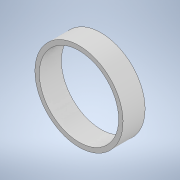
# Autodesk Inventor part: 轴承盖挡圈
Saved by Autodesk Inventor 2020 (Build 240168000, 168)
## iProperties
Created: 2021-06-16
Part Number: 轴承盖挡圈
Material: 常规
Document SubType Name: Modeling
Designer: dell
Density: 1 g/cm^3
Appearance: 默认
Author: dell
Autodesk Inventor part; units mm, degrees
ref_plane "YZ Plane" through (0, 0, 0) normal (1, 0, 0) x (0, 1, 0)
ref_plane "XZ Plane" through (0, 0, 0) normal (0, 1, 0) x (-1, 0, 0)
ref_plane "工作平面1" through (-16.8643, 32.5395, 28) normal (0, 0, 1) x (-0.4601, 0.8878, 0)
sketch "草图1" plane through (-16.8643, 32.5395, 28) normal (0, 0, 1) x (-0.4601, 0.8878, 0)
  circle A0 centre (-36.65, 0) radius 65 construction
  circle A1 centre (-36.65, 0) radius 40
  circle A2 centre (-36.65, 0) radius 32
  point P0 (-36.65, 0)
  dimension "d0" = 80
  dimension "d1" = 64
  constraints: 2 centre point, 2 coincident
  measures "d0" diameter of A1
  measures "d1" diameter of A2
extrude "拉伸1" add sketch "草图1" along normal blind 20
sketch "草图2" plane through (0, 0, 48) normal (0, 0, 1) x (1, 0, 0)
  circle A0 centre (0, 0) radius 36
  dimension "d4" = 72
  constraints: 1 centre point, 1 coincident
  measures "d4" diameter of A0
extrude "拉伸2" cut sketch "草图2" against normal up to surface (20 mm away)
